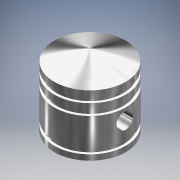
# Autodesk Inventor part: piston
Saved by Autodesk Inventor 2018.1 (Build 221171000, 171)
## iProperties
Created: 2013-08-27
Part Number: piston
Material: Generic
Document SubType Name: Modeling
Designer: Konstantin
Density: 1 g/cm^3
Appearance: Default
Mass: 0.751299 g
Surface Area: 12.0212 cm^2
Volume: 0.751299 cm^3
Author: Konstantin
Autodesk Inventor part; units mm, degrees
ref_plane "YZ Plane" through (0, 0, 0) normal (1, 0, 0) x (0, 1, 0)
ref_plane "XY Plane" through (0, 0, 0) normal (0, 0, 1) x (1, 0, 0)
sketch "Sketch1" plane through (0, 0, 0) normal (0, 0, 1) x (1, 0, 0)
  line L0 (5, 0) -> (6.45, 0)
  line L1 (0, 13) -> (0, 11.4819)
  line L2 (6, 1) -> (6.45, 1)
  line L3 (6, 1.8) -> (6.45, 1.8)
  line L4 (6, 1.8) -> (6, 1)
  line L5 (6.45, 0) -> (6.45, 1)
  line L6 (6, 7) -> (6.45, 7)
  line L7 (6, 7.8) -> (6.45, 7.8)
  line L8 (6, 7.8) -> (6, 7)
  line L9 (6.45, 1.8) -> (6.45, 7)
  line L10 (6, 9) -> (6.45, 9)
  line L11 (6, 9.8) -> (6.45, 9.8)
  line L12 (6, 9.8) -> (6, 9)
  line L13 (6.45, 7.8) -> (6.45, 9)
  line L14 (6.45, 9.8) -> (6.45, 11)
  line L15 (0, 13) -> (6.45, 11)
  line L16 (5, 9.9315) -> (5, 0)
  line L17 (0, 11.4819) -> (5, 9.9315)
  point P0 (0, 0)
  constraints: 36 end point, 9 parallel, 9 vertical, 8 horizontal, 8 perpendicular, 2 other
revolve "Revolution1" add sketch "Sketch1" angle 360 about axis through (0, 13, 0) along (0, -1, 0)
ref_plane "Work Plane1" through (0, 2, 0) normal (0, 1, 0) x (-1, 0, 0)
sketch "Sketch2" plane through (0, 2, 0) normal (0, 1, 0) x (-1, 0, 0)
  line L0 (-3, 2.5) -> (-3, -2.5)
  line L1 (3, 2.5) -> (3, -2.5)
  line L2 (4.3301, 2.5) -> (3, 2.5)
  line L3 (-3, 2.5) -> (-4.3301, 2.5)
  line L4 (4.3301, -2.5) -> (3, -2.5)
  line L5 (-3, -2.5) -> (-4.3301, -2.5)
  arc A0 (-4.3301, 2.5) -> (-4.3301, -2.5) centre (0, 0) ccw
  arc A1 (4.3301, -2.5) -> (4.3301, 2.5) centre (0, 0) ccw
  constraints: 12 end point, 5 parallel, 4 horizontal, 4 point on circle, 2 centre point, 2 vertical, 2 other
extrude "Extrusion1" add sketch "Sketch2" along normal blind 9
fillet "Fillet1" radius 2.5 4 edges at (-3.6651, 2, 2.5) (-3.6651, 2, -2.5) (3.6651, 2, 2.5) (3.6651, 2, -2.5)
sketch "Sketch3" plane through (0, 0, 0) normal (1, 0, 0) x (0, 1, 0)
  circle A0 centre (5, 0) radius 1.5
  constraints: 1 centre point, 1 other
extrude "Extrusion2" cut sketch "Sketch3" along normal mid plane 20
body "Solid1"
